lego-tray-corner-left (Autodesk Fusion 360 design; units mm, degrees)
Autodesk Fusion 360 part; units mm, degrees
note: some values were not read from the file. Set by a fixed rule: which sketch regions a step uses.
sketch "Sketch1" plane through (0, 0, 0) normal (0, 1, 0) x (1, 0, 0)
  line L0 (0, 0) -> (-82.2706, 0)
  line L1 (-82.2706, 0) -> (-82.2706, 65.5066)
  line L2 (-20.3962, 127.381) -> (0, 127.381)
  line L3 (0, 127.381) -> (0, 0)
  arc A0 (-20.3962, 127.381) -> (-82.2706, 65.5066) centre (-20.3962, 65.5066) ccw
  line L4 (-81.8896, 0.381) -> (-81.8896, 65.5066)
  arc A1 (-20.3962, 127) -> (-81.8896, 65.5066) centre (-20.3962, 65.5066) ccw
  line L5 (-20.3962, 127) -> (-0.381, 127)
  line L6 (-0.381, 127) -> (-0.381, 0.381)
  line L7 (-0.381, 0.381) -> (-81.8896, 0.381)
  dimension "d1" = 82.2706
  dimension "d2" = 127.381
  dimension "d3" = 61.8744
  dimension "d23" = -0.381
  constraint horizontal L0
  constraint vertical L1
  constraint horizontal L2
  constraint vertical L3
  constraint coincident L0.start L3.end
  constraint tangent L1 A0
  constraint tangent L2 A0
  measures "d1" distance of L0.start L0.end
  measures "d2" distance of L0.start L2.end
  measures "d3" radius of A0
extrude "Extrude1" add sketch "Sketch1" along normal blind 76.2 contours L4 A1 L5 L6 L7
draft "Draft1" angle -4 neutral plane through (0, 0, 0) pull (0, 1, 0) 3 faces at (-81.8896, 25.4, -22.0895) (-81.8199, 50.8, -68.4326) (-13.7245, 25.4, -127)
fillet "Fillet1" radius 6.35 3 edges at (-0.381, 38.1, -129.6642) (-84.5538, 38.1, -0.381) (-0.381, 38.1, -0.381)
fillet "Fillet2" radius 3.175 8 edges at (-2.2409, 0, -2.2409) (-41.1275, 0, -0.381) (-80.0252, 0, -2.2409) (-81.8896, 0, -36.1188) (-63.8786, 0, -108.989) (-13.5636, 0, -127) (-2.2409, 0, -125.1356) (-0.381, 0, -63.6827)
shell "Shell1" thickness 1.524 removed faces 1 at (-28.4244, 76.2, -72.3421)
sketch "Sketch2" plane through (0, 76.2, 0) normal (0, 1, 0) x (-1, 0, 0)
  line L0 (68.1525, -0.381) -> (49.1025, -0.381)
  line L1 (49.1025, -0.381) -> (49.1025, -1.905)
  line L2 (49.1025, -1.905) -> (68.1525, -1.905)
  line L3 (68.1525, -1.905) -> (68.1525, -0.381)
  line L4 (1.905, -19.431) -> (0.381, -19.431)
  line L5 (0.381, -19.431) -> (0.381, -63.881)
  line L6 (0.381, -63.881) -> (1.905, -63.881)
  line L7 (1.905, -63.881) -> (1.905, -19.431)
  line L8 (0.381, -6.731) -> (0.381, -125.9629)
  line L9 (1.905, -125.9629) -> (1.905, -6.731)
  line L10 (6.731, -1.905) -> (80.8525, -1.905)
  line L11 (80.8525, -0.381) -> (6.731, -0.381)
  dimension "d14" = 44.45
  dimension "d15" = 19.05
  dimension "d28" = 12.7
  dimension "d29" = 12.7
  constraint horizontal L0
  constraint vertical L1
  constraint horizontal L2
  constraint vertical L3
  constraint horizontal L4
  constraint vertical L5
  constraint horizontal L6
  constraint vertical L7
  constraint coincident L2.end L10
  constraint coincident L0.end L11
  constraint coincident L6.end L9
  constraint coincident L4.end L8
  measures "d14" distance of L4.end L5.end
  measures "d15" distance of L0.start L0.end
  measures "d28" distance of L0.start L11.start
  measures "d29" distance of L4.end L8.start
extrude "Extrude2" cut sketch "Sketch2" against normal blind 12.7
draft "Draft2" angle 30 neutral plane through (0, 63.5, 0) pull (0, 1, 0) 4 faces at (-49.1025, 67.7333, -0.889) (-0.889, 67.7333, -63.881) (-1.397, 67.7333, -19.431) (-68.1525, 67.7333, -1.397)
fillet "Fillet3" radius 6.35 8 edges at (-75.4849, 76.2, -1.143) (-68.1525, 63.5, -1.143) (-41.7702, 76.2, -1.143) (-49.1025, 63.5, -1.143) (-1.143, 76.2, -12.0987) (-1.143, 63.5, -19.431) (-1.143, 63.5, -63.881) (-1.143, 76.2, -71.2133)
